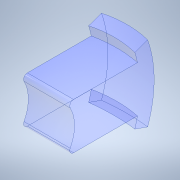
# Autodesk Inventor part: shank_2
Saved by Autodesk Inventor 2020.2 (Build 242310000, 310)
## iProperties
Created: 2021-01-30
Part Number: shank_2
Material: Generic
Document SubType Name: Modeling
Designer: DELL
Density: 1 g/cm^3
Appearance: Clear - Blue
Author: DELL
Autodesk Inventor part; units mm, degrees
ref_plane "XZ Plane" through (0, 0, 0) normal (0, 1, 0) x (-1, 0, 0)
ref_plane "XY Plane" through (0, 0, 0) normal (0, 0, 1) x (1, 0, 0)
ref_plane "UCS1: YZ Plane" through (0, 0, 0) normal (1, 0, 0) x (0, 1, 0)
sketch "Sketch17" plane through (0, 0, 0) normal (1, 0, 0) x (0, 1, 0)
  line L0 (-112, 0) -> (112, 0) construction
  line L1 (0, -195.7) -> (0, 89.2) projected
  circle A0 centre (0, 0) radius 40
  circle A1 centre (0, 0) radius 48.5
  arc A2 (-72.2892, -117.8664) -> (72.2892, -117.8664) centre (0, 13.5652) ccw
  arc A3 (-80, -131.8858) -> (80, -131.8858) centre (0, -5) ccw
  line L2 (72.2892, -117.8664) -> (80, -131.8858)
  line L3 (-80, -131.8858) -> (-72.2892, -117.8664)
  line L4 (-30, -38.1084) -> (-30, -136.4348)
  line L5 (-30, -136.4348) -> (30, -136.4348)
  line L6 (30, -136.4348) -> (30, -38.1084)
  line L7 (-44.1229, -129.7985) -> (-50, -146.4214)
  line L8 (44.1229, -129.7985) -> (50, -146.4214)
  point P0 (0, -155)
  point P1 (0, -136.4348)
  point P2 (0, -155)
  dimension "d173" = 97
  dimension "d174" = 80
  dimension "d224" = 60
  dimension "d229" = 155
  dimension "d230" = 150
  dimension "d231" = 16
  dimension "d232" = 100
  dimension "d233" = 30
  dimension "d235" = 150
  constraints: 14 end point, 12 point on circle, 4 centre point, 2 coincident, 2 line through centre, 2 perpendicular, 2 point on line, 1 tangent, 1 vertical, 3 other
  measures "d173" diameter of A1
  measures "d174" diameter of A0
  measures "d224" distance of L4.end L5.end
  measures "d229" distance from line of point (0, -155) L0
  measures "d230" radius of A3
  measures "d231" distance of L2.start L2.end
  measures "d232" diameter of L7.end L1
  measures "d233" horizontal distance of L3.start L7.end
  measures "d235" radius of A2
sketch "Sketch16" plane through (0, 0, 0) normal (1, 0, 0) x (0, 1, 0)
  circle A0 centre (0, 0) radius 40
  circle A1 centre (0, 0) radius 48.5
  line L0 (0, -201.7) -> (0, 90.2) construction
  line L1 (0, -160) -> (0, -48.5)
  line L2 (30, -38.1084) -> (30, -103.6436)
  line L3 (30, -103.6436) -> (25, -132)
  line L4 (25, -132) -> (50, -132)
  line L5 (50, -132) -> (50, -160)
  line L6 (50, -160) -> (0, -160)
  dimension "d156" = 97
  dimension "d157" = 80
  dimension "d202" = 28
  dimension "d203" = 60
  dimension "d204" = 50
  dimension "d206" = 160
  dimension "d209" = 50
  dimension "d210" = 80
  dimension "d211" = 28.7938
  constraints: 12 end point, 2 centre point, 2 coincident, 2 horizontal, 2 point on circle, 2 point on line, 2 vertical
  measures "d156" diameter of A1
  measures "d157" diameter of A0
  measures "d202" distance of L4.end L5.end
  measures "d203" diameter of L2 L0
  measures "d204" distance of L5.end L1.start
  measures "d206" distance from line of point (0, 0) L6
  measures "d209" diameter of L3.end L0
  measures "d210" angle of L4 L3
  measures "d211" distance of L2.end L3.end
extrude "Extrusion14" [suppressed]
fillet "Fillet10" [suppressed]
mirror "Mirror1" [suppressed]
thicken "Thicken1" [suppressed]
sketch "Sketch19" plane through (0, 0, 0) normal (0, 1, 0) x (-1, 0, 0)
  arc A0 (-110.8458, -111.0605) -> (110.8458, -111.0605) centre (0, -10) ccw
  line L0 (155.1841, 0) -> (-155.1841, 0) projected
  line L1 (0, -264.129) -> (0, 44.0215) projected
  line L2 (110.8458, -111.0605) -> (110.8458, -220.1075)
  line L3 (110.8458, -220.1075) -> (-110.8458, -220.1075)
  line L4 (-110.8458, -220.1075) -> (-110.8458, -111.0605)
  point P0 (0, 0)
  point P1 (0, -160)
  point P2 (0, -160)
  point P3 (0, -220.1075)
  dimension "d217" = 150
  dimension "d218" = 0
  constraints: 6 end point, 3 point on circle, 2 point on line, 2 vertical, 1 centre point, 1 horizontal, 1 symmetric about line
  measures "d217" radius of A0
  measures "d218" distance of point (0, -160) point (0, -160)
revolve "Revolution1" [suppressed]
fillet "Fillet15" [suppressed]
revolve "Revolution2" add sketch "Sketch17" angle 360 about axis through (0, 0, -10) along (0, 0, 1) separate body contours L1 L5 L6 A2 L8 A3 | A2 L6 L5 | L8 A2 L2 A3
ref_plane "Work Plane7" through (0, -44.1229, -129.7985) normal (0, -0.942809, 0.3333333) x (0, -0.3333333, -0.942809)
split "Split2" plane through (0, -44.1229, -129.7985) removes the side toward (0, -0.942809, 0.3333333)
ref_plane "Work Plane8" through (0, 44.1229, -129.7985) normal (0, -0.942809, -0.3333333) x (0, 0.3333333, -0.942809)
split "Split3" plane through (0, 44.1229, -129.7985) removes the side toward (0, 0.942809, 0.3333333)
ref_plane "Work Plane9" through (-30, 0, 0) normal (1, 0, 0) x (0, 1, 0)
split "Split4" plane through (-30, 0, 0) removes the side toward (-1, 0, 0)
ref_plane "Work Plane10" through (30, 0, 0) normal (1, 0, 0) x (0, 1, 0)
split "Split5" plane through (30, 0, 0) removes the side toward (1, 0, 0)
extrude "Extrusion17" add sketch "Sketch17" along normal mid plane 60 contours A2 L4 A1 L1 | L5 L4 A2 | L1 A1 L6 A2 | A2 L6 L5
fillet "Fillet16" radius 5 2 edges at (0, 30, -38.1084) (0, -30, -38.1084)
body "Solid1"
body "Solid6"
body "Solid8"
